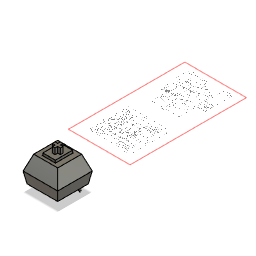
Key switch v2 (Autodesk Fusion 360 design; units mm, degrees)
Autodesk Fusion 360 part; units mm, degrees
sketch "Sketch1" plane through (0, 0, 0) normal (0, 1, 0) x (1, 0, 0)
sketch "Sketch2" plane through (0, 0, 0) normal (0, 1, 0) x (1, 0, 0)
sketch "Sketch3" plane through (0, 0, 0) normal (0, 1, 0) x (1, 0, 0)
  line L0 (-7.8, -52.8) -> (7.8, -52.8)
  line L1 (7.8, -52.8) -> (7.8, -37.2)
  line L2 (7.8, -37.2) -> (-7.8, -37.2)
  line L3 (-7.8, -37.2) -> (-7.8, -52.8)
  line L4 (-7.8, -52.8) -> (7.8, -37.2) construction
  line L5 (7.8, -52.8) -> (-7.8, -37.2) construction
  point P0 (0, -45)
  dimension "d3" = 15.6
  dimension "d4" = 15.6
  constraint horizontal L0
  constraint perpendicular L0 L1
  constraint parallel L0 L2
  constraint parallel L1 L3
  constraint coincident L4 P0
  constraint coincident L5 P0
  measures "d3" distance of L1.end L2.end
  measures "d4" distance of L0.end L1.end
extrude "Extrude1" add sketch "Sketch3" along normal blind 6.6 draft -20 makes body 1
sketch "Sketch4" plane through (0, 0, 0) normal (1, 0, 0) x (0, 0, -1)
extrude "Extrude2" add 1 faces at (-2.6, 0, 42.4) along direction (0, -1, 0) blind 5 draft -10 on bodies 1 bodies 1
sketch "Sketch5" plane through (0, 6.6, 0) normal (0, 1, 0) x (-1, 0, 0)
  line L0 (-5.3978, 39.6022) -> (5.3978, 39.6022)
  line L1 (5.3978, 39.6022) -> (5.3978, 50.3978)
  line L2 (5.3978, 50.3978) -> (-5.3978, 50.3978)
  line L3 (-5.3978, 50.3978) -> (-5.3978, 39.6022)
  line L4 (-3, 41) -> (3, 41)
  line L5 (3, 41) -> (3, 49)
  line L6 (3, 49) -> (-3, 49)
  line L7 (-3, 49) -> (-3, 41)
  line L8 (-3, 41) -> (3, 49) construction
  line L9 (3, 41) -> (-3, 49) construction
  point P0 (0, 45)
  constraint horizontal L4
  constraint perpendicular L4 L5
  constraint parallel L4 L6
  constraint parallel L5 L7
  constraint coincident L8 P0
  constraint coincident L9 P0
extrude "Extrude3" cut sketch "Sketch5" against normal blind 1 contours L4 L5 L6 L7 bodies 1
sketch "Sketch6" plane through (0, 5.6, 0) normal (0, 1, 0) x (-1, 0, 0)
  line L0 (-3, 49) -> (-3, 41)
  line L1 (-3, 41) -> (3, 41)
  line L2 (3, 41) -> (3, 49)
  line L3 (3, 49) -> (-3, 49)
  line L4 (2.8, 41.1) -> (-2.8305, 41.1)
  line L5 (-2.8305, 41.1) -> (-2.8305, 48.9)
  line L6 (-2.8305, 48.9) -> (2.8, 48.9)
  line L7 (2.8, 48.9) -> (2.8, 41.1)
  line L8 (2.8, 41.1) -> (-2.8305, 48.9) construction
  line L9 (-2.8305, 41.1) -> (2.8, 48.9) construction
  point P0 (-0.0152, 45)
  constraint horizontal L4
  constraint perpendicular L4 L5
  constraint parallel L4 L6
  constraint parallel L5 L7
  constraint coincident L8 P0
  constraint coincident L9 P0
extrude "Extrude4" add sketch "Sketch6" along normal blind 2 contours L4 L5 L6 L7 bodies 1
sketch "Sketch7" plane through (0, 7.6, 0) normal (0, 1, 0) x (-1, 0, 0)
  line L0 (2.8, 48.9) -> (-2.8305, 48.9)
  line L1 (-2.8305, 48.9) -> (-2.8305, 41.1)
  line L2 (-2.8305, 41.1) -> (2.8, 41.1)
  line L3 (2.8, 41.1) -> (2.8, 48.9)
  line L4 (0.6, 43.2) -> (-0.6, 43.2)
  line L5 (-0.6, 43.2) -> (-0.6, 46.8)
  line L6 (-0.6, 46.8) -> (0.6, 46.8)
  line L7 (0.6, 46.8) -> (0.6, 43.2)
  line L8 (0.6, 43.2) -> (-0.6, 46.8) construction
  line L9 (-0.6, 43.2) -> (0.6, 46.8) construction
  line L10 (-1.8, 44.4) -> (1.8, 44.4)
  line L11 (1.8, 44.4) -> (1.8, 45.6)
  line L12 (1.8, 45.6) -> (-1.8, 45.6)
  line L13 (-1.8, 45.6) -> (-1.8, 44.4)
  line L14 (-1.8, 44.4) -> (1.8, 45.6) construction
  line L15 (1.8, 44.4) -> (-1.8, 45.6) construction
  point P0 (0, 45)
  point P1 (0, 45)
  constraint horizontal L4
  constraint perpendicular L4 L5
  constraint parallel L4 L6
  constraint parallel L5 L7
  constraint coincident L8 P1
  constraint coincident L9 P1
  constraint horizontal L10
  constraint perpendicular L10 L11
  constraint parallel L10 L12
  constraint parallel L11 L13
  constraint coincident L14 P1
  constraint coincident L15 P1
  constraint coincident P1 P0
extrude "Extrude5" add sketch "Sketch7" along normal blind 3.2 contours L4 L5 L7 L10 | L5 L7 L10 L12 | L7 L10 L11 L12 | L5 L10 L12 L13 | L5 L6 L7 L12 bodies 1
sketch "Sketch8" plane through (-2.8, 0, 0) normal (-1, 0, 0) x (0, 0, 1)
  line L0 (41.1, 5.6) -> (48.9, 5.6)
  line L1 (48.9, 5.6) -> (48.9, 7.6)
  line L2 (48.9, 7.6) -> (41.1, 7.6)
  line L3 (41.1, 7.6) -> (41.1, 5.6)
extrude "Extrude6" cut 1 faces at (1.4, 10.8, 45.2) along direction (0, -1, 0) blind 0.6 on bodies 1 bodies 1
sketch "Sketch9" plane through (0, -5, 0) normal (0, -1, 0) x (1, 0, 0)
  line L0 (6.9184, 51.9184) -> (-6.9184, 51.9184)
  line L1 (-6.9184, 51.9184) -> (-6.9184, 38.0816)
  line L2 (-6.9184, 38.0816) -> (6.9184, 38.0816)
  line L3 (6.9184, 38.0816) -> (6.9184, 51.9184)
  circle A0 centre (0, 45) radius 3
extrude "Extrude7" add sketch "Sketch9" along normal blind 2.5 contours A0 bodies 1
extrude "Extrude8" add 1 faces at (0.8808, -7.5, 44.8347) along direction (0, -1, 0) blind 0.8 draft -45 on bodies 1 bodies 1
sketch "Sketch10" plane through (0, -5, 0) normal (0, -1, 0) x (1, 0, 0)
  circle A0 centre (0, 45) radius 3
  line L0 (6.9184, 51.9184) -> (-6.9184, 51.9184)
  line L1 (-6.9184, 51.9184) -> (-6.9184, 38.0816)
  line L2 (-6.9184, 38.0816) -> (6.9184, 38.0816)
  line L3 (6.9184, 38.0816) -> (6.9184, 51.9184)
  circle A1 centre (-5, 42.5) radius 0.5
  circle A2 centre (5, 40) radius 0.5
extrude "Extrude9" add sketch "Sketch10" along normal blind 2.5 contours A1 | A2 bodies 1
extrude "Extrude10" add 2 faces at (-5.0609, -7.5, 42.6551) (4.9391, -7.5, 40.1551) along direction (0, -1, 0) blind 0.8 draft -25 on bodies 1 bodies 1
sketch "Sketch11" plane through (-2.8, 0, 0) normal (-1, 0, 0) x (0, 0, 1)
copy_body "Body->Comp1" bodies 1 removing the originals makes body 2 in component "Switch"
component "Switch" placed x (1, 0, 0) y (0, 1, 0) z (0, 0, 1) at (0, 0, 0)
